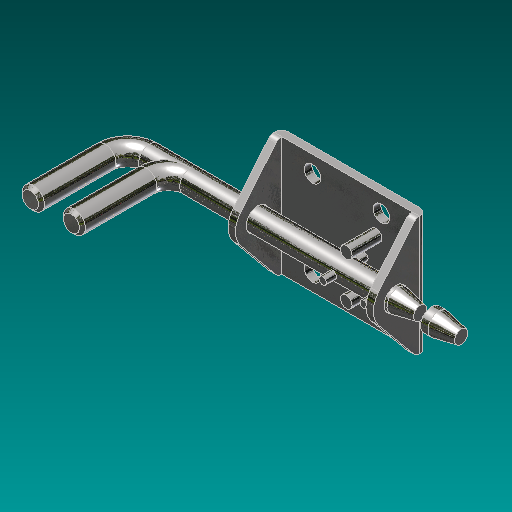
# Autodesk Inventor part: Spring latch
Saved by Autodesk Inventor 2017 (Build 210142000, 142)
## iProperties
Created: 2013-06-17
Part Number: Spring latch
Material: Steel, Galvanized
Document SubType Name: Modeling
Designer: Graeme_Van_Dongen
Density: 7.85 g/cm^3
Appearance: Galvanized
Mass: 216.104 g
Surface Area: 161.001 cm^2
Volume: 27.5292 cm^3
Author: Graeme_Van_Dongen
Autodesk Inventor part; units mm, degrees
ref_plane "YZ Plane" through (0, 0, 0) normal (1, 0, 0) x (0, 1, 0)
ref_plane "XZ Plane" through (0, 0, 0) normal (0, 1, 0) x (-1, 0, 0)
ref_plane "XY Plane" through (0, 0, 0) normal (0, 0, 1) x (1, 0, 0)
sketch "Sketch1" plane through (0, 0, 0) normal (0, 0, 1) x (1, 0, 0)
  line L0 (-30.9562, -25.4) -> (30.9563, -25.4)
  line L1 (30.9563, -25.4) -> (30.9562, 25.4)
  line L2 (30.9562, 25.4) -> (-30.9563, 25.4)
  line L3 (-30.9563, 25.4) -> (-30.9562, -25.4)
  line L4 (-30.9562, -25.4) -> (30.9562, 25.4) construction
  point P0 (0, 0)
  point P1 (0, 0)
  dimension "d0" = 61.9125
  dimension "d1" = 50.8
  constraints: 10 end point, 2 parallel, 1 coincident, 1 horizontal, 1 midpoint, 1 perpendicular
  measures "d0" distance of L2.end L1.end
  measures "d1" distance of L1.end L0.end
extrude "Extrusion1" add sketch "Sketch1" along normal blind 25.4
sketch "Sketch2" plane through (30.9563, -25.4, 0) normal (1, 0, 0) x (0, 0, -1)
  line L0 (0, 0) -> (0, 50.8) projected
  line L1 (0, 0) -> (-3.175, 0)
  arc A0 (-5.6204, 1.15) -> (-3.175, 0) centre (-3.175, 3.175) ccw
  line L2 (-5.6204, 1.15) -> (-20.6711, 19.3249)
  arc A1 (-20.6711, 31.4751) -> (-20.6711, 19.3249) centre (-13.335, 25.4) ccw
  line L3 (-20.6711, 31.4751) -> (-5.6204, 49.65)
  arc A2 (-3.175, 50.8) -> (-5.6204, 49.65) centre (-3.175, 47.625) ccw
  line L4 (-3.175, 50.8) -> (0, 50.8)
  point P0 (0, 25.4)
  point P1 (0, 25.4)
  point P2 (0, 25.4)
  dimension "d4" = 3.175
  dimension "d5" = 3.175
  dimension "d6" = 22.86
  dimension "d7" = 9.525
  constraints: 8 end point, 6 point on circle, 6 tangent, 3 centre point, 2 equal length, 2 midpoint, 1 equal radius, 1 horizontal alignment, 1 parallel, 1 perpendicular
  measures "d4" distance of L0.start L1.end
  measures "d5" radius of A0
  measures "d7" radius of A1
extrude "Extrusion2" cut sketch "Sketch2" against normal through all keep common part
shell "Shell1" thickness 3.175 removed faces 5 at (-10.3187, -24.9916, 4.7328) at (-10.3187, -12.1334, 15.6542) at (10.3187, 12.1334, 15.6542) at (-10.3188, 24.8701, 4.9311) at (10.3187, 5.4939, 21.1159)
fillet "Fillet1" radius 3.175 2 edges at (-30.9563, 0, 0) (30.9562, 0, 0)
hole "Hole1" at (30.9562, 0, 13.335) direction (-1, 0, 0) diameter 9.9219 end through all
sketch "Sketch3" plane through (0, 0, 0) normal (0, 0, -1) x (-1, 0, 0)
  line L0 (14.6844, 18.2563) -> (-14.6844, 18.2562)
  line L1 (-14.6844, 18.2562) -> (-14.6844, -18.2563)
  line L2 (-14.6844, -18.2563) -> (14.6844, -18.2562)
  line L3 (14.6844, -18.2562) -> (14.6844, 18.2563)
  line L4 (14.6844, 18.2563) -> (-14.6844, -18.2563)
  point P0 (0, 0)
  point P1 (0, 0)
  dimension "d21" = 29.3687
  dimension "d22" = 36.5125
  constraints: 10 end point, 5 coincident, 2 parallel, 1 horizontal, 1 midpoint, 1 perpendicular
  measures "d21" distance of L2.end L1.end
  measures "d22" distance of L0.end L1.end
hole "Hole2" at (-14.6844, -18.2562, 0) at (-14.6844, 18.2563, 0) at (14.6844, 18.2562, 0) at (14.6844, -18.2563, 0) direction (0, 0, 1) diameter 7.0358 end through all
sketch "Sketch4" plane through (0, 0, 0) normal (0, 1, 0) x (-1, 0, 0)
  line L0 (-30.9563, 8.3741) -> (-30.9563, 18.2959) construction
  line L1 (30.9563, 18.2959) -> (30.9563, 8.3741) construction
  line L2 (-58.8963, 13.335) -> (56.3562, 13.335)
  arc A0 (56.3562, 13.335) -> (65.8812, 22.86) centre (56.3563, 22.86) ccw
  line L3 (65.8812, 22.86) -> (65.8812, 54.61)
  point P0 (0, 0)
  point P1 (30.9563, 13.335)
  dimension "d30" = 27.94
  dimension "d31" = 34.925
  dimension "d32" = 9.525
  dimension "d33" = 41.275
  constraints: 4 end point, 2 perpendicular, 2 point on circle, 2 tangent, 1 centre point, 1 midpoint, 1 point on line
  measures "d30" distance from line of L0 L2.start
  measures "d31" distance between parallel lines of L1 L3
  measures "d32" radius of A0
  measures "d33" distance from line of L2 L3.end
sketch "Sketch5" plane through (0, 0, 0) normal (1, 0, 0) x (0, 1, 0)
  circle A0 centre (0, 13.335) radius 4.7117
  point P0 (0, 0)
  point P1 (0, 13.335)
  dimension "d34" = 9.4234
  constraints: 1 centre point, 1 coincident
  measures "d34" diameter of A0
sweep "Sweep1" add profiles "Sketch5" path "Sketch4"
chamfer "Chamfer1" distance 1.27 angle 45 1 edges at (-65.8813, -4.7117, 54.61)
chamfer "Chamfer2" distance 9.525 angle 11 1 edges at (58.8963, -4.7117, 13.335) measured on face at (58.3963, -4.7117, 13.335)
sketch "Sketch6" plane through (-27.7812, -25.4, 3.175) normal (0, 0, 1) x (1, 0, 0)
  circle A0 centre (40.2101, 16.2719) radius 2.5
  circle A1 centre (40.2101, 34.5281) radius 2.5
  line L0 (40.2101, 34.5281) -> (40.2101, 16.2719) construction
  line L1 (27.7812, 25.4) -> (40.2101, 25.4) construction
  line L2 (55.5625, 0) -> (55.5625, 50.8) construction
  dimension "d42" = 5
  dimension "d44" = 12.8524
  dimension "d45" = 18.2563
  constraints: 4 end point, 2 centre point, 1 equal radius, 1 midpoint, 1 perpendicular, 1 vertical
  measures "d42" diameter of A1
  measures "d44" distance edge to line of A1 L2
  measures "d45" distance of L0.start L0.end
extrude "Extrusion3" add sketch "Sketch6" along normal blind 12.7
ref_plane "Work Plane1" through (58.8963, 0, 13.335) normal (0, 0, -1) x (-1, 0, 0)
sketch "Sketch7" plane through (58.8963, 0, 13.335) normal (0, 0, -1) x (-1, 0, 0)
  circle A0 centre (32.7025, 0) radius 1.5875
  line L0 (31.115, -25.4) -> (31.115, 25.4) construction
  point P0 (58.8963, 0)
  dimension "d49" = 3.175
  constraints: 1 centre point, 1 horizontal alignment, 1 tangent
  measures "d49" diameter of A0
extrude "Extrusion4" add sketch "Sketch7" along normal mid plane 17.78
pattern_linear "Rectangular Pattern1" count 2 spacing 17.4625 along (-1, 0, 0) of "Sweep1", "Chamfer1", "Extrusion4"
sketch "Sketch8" plane through (58.8963, 0, 13.335) normal (0, 0, -1) x (-1, 0, 0)
  line L0 (0, -2.8602) -> (0, 2.8602) construction
  line L1 (12.7, -4.7117) -> (17.4625, -4.7117)
  line L2 (17.4625, -4.7117) -> (17.4625, 4.7117)
  line L3 (17.4625, 4.7117) -> (12.7, 4.7117)
  line L4 (12.7, 4.7117) -> (12.7, -4.7117)
  line L5 (9.525, 4.7117) -> (132.715, 4.7117) construction
  line L6 (9.525, -4.7117) -> (132.715, -4.7117) construction
  point P0 (58.8963, 0)
  dimension "d55" = 12.7
  dimension "d56" = 17.4625
  constraints: 8 end point, 2 collinear, 2 parallel, 1 horizontal, 1 perpendicular
  measures "d55" distance between parallel lines of L0 L4
  measures "d56" distance between parallel lines of L0 L2
extrude "Extrusion5" cut sketch "Sketch8" along normal through all both and the other way through all
chamfer "Chamfer3" distance 9.525 angle 11 1 edges at (41.4338, -4.7117, 13.335) measured on face at (40.9338, -4.7117, 13.335)
equation "\"d56\" = d54"
equation "\"d59\" = d39"
equation "\"d61\" = d41"
equation "\"d54\" = 17.4625"
equation "\"d39\" = 9.525"
equation "\"d41\" = 11deg"
body "Solid1"
